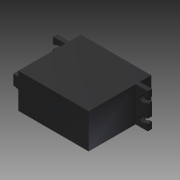
# Autodesk Inventor part: servo 4.8kg TGY-S4505B
Saved by Autodesk Inventor 2013 (Build 170138000, 138)
## iProperties
Created: 2013-03-06
Part Number: servo 4.8kg TGY-S4505B
Material: Generic
Document SubType Name: Modeling
Designer: Masta
Density: 1 g/cm^3
Author: Masta
Autodesk Inventor part; units mm, degrees
ref_plane "YZ Plane" through (0, 0, 0) normal (1, 0, 0) x (0, 1, 0)
ref_plane "XZ Plane" through (0, 0, 0) normal (0, 1, 0) x (-1, 0, 0)
ref_plane "XY Plane" through (0, 0, 0) normal (0, 0, 1) x (1, 0, 0)
sketch "Sketch1" plane through (0, 0, 0) normal (0, 1, 0) x (-1, 0, 0)
  line L0 (20.25, 10) -> (-20.25, 10)
  line L1 (-20.25, 10) -> (-20.25, -10)
  line L2 (-20.25, -10) -> (20.25, -10)
  line L3 (20.25, -10) -> (20.25, 10)
  line L4 (20.25, 10) -> (-20.25, -10) construction
  line L5 (-20.25, 10) -> (20.25, -10) construction
  line L6 (-27.25, 10) -> (-27.25, 6.25)
  line L7 (27.25, -10) -> (27.25, -6.25)
  line L8 (27.25, 10) -> (-27.25, -10) construction
  line L9 (-27.25, 10) -> (27.25, -10) construction
  line L10 (20.25, -10) -> (27.25, -10)
  line L11 (20.25, 10) -> (27.25, 10)
  line L12 (-20.25, 10) -> (-27.25, 10)
  line L13 (-20.25, -10) -> (-27.25, -10)
  line L14 (24.25, 5) -> (-24.25, 5) construction
  line L15 (-24.25, 5) -> (-24.25, -5) construction
  line L16 (-24.25, -5) -> (24.25, -5) construction
  line L17 (24.25, -5) -> (24.25, 5) construction
  line L18 (24.25, 5) -> (-24.25, -5) construction
  line L19 (-24.25, 5) -> (24.25, -5) construction
  circle A0 centre (-24.25, 5) radius 2
  line L20 (-27.25, 3.75) -> (-25.8112, 3.75)
  line L21 (-27.25, 6.25) -> (-25.8112, 6.25)
  line L22 (-20.25, 0) -> (20.25, 0) construction
  line L23 (0, 10) -> (0, -10) construction
  circle A1 centre (-24.25, -5) radius 2
  line L24 (-27.25, -3.75) -> (-25.8112, -3.75)
  line L25 (-27.25, -6.25) -> (-25.8112, -6.25)
  circle A2 centre (24.25, 5) radius 2
  line L26 (27.25, 3.75) -> (25.8112, 3.75)
  line L27 (27.25, 6.25) -> (25.8112, 6.25)
  line L28 (27.25, -6.25) -> (25.8112, -6.25)
  line L29 (27.25, -3.75) -> (25.8112, -3.75)
  circle A3 centre (24.25, -5) radius 2
  line L30 (-27.25, 3.75) -> (-27.25, -3.75)
  line L31 (-27.25, 6.25) -> (-27.25, 3.75)
  line L32 (-27.25, -6.25) -> (-27.25, -10)
  line L33 (-27.25, -3.75) -> (-27.25, -6.25)
  line L34 (27.25, -3.75) -> (27.25, 3.75)
  line L35 (27.25, -6.25) -> (27.25, -3.75)
  line L36 (27.25, 3.75) -> (27.25, 6.25)
  line L37 (27.25, 6.25) -> (27.25, 10)
  point P0 (0, 0)
  dimension "d0" = 40.5
  dimension "d1" = 20
  dimension "d2" = 54.5
  dimension "d3" = 48.5
  dimension "d4" = 10
  dimension "d12" = 2.5
  dimension "d13" = 4
  constraints: 76 end point, 32 parallel, 15 symmetric about line, 12 perpendicular, 10 midpoint, 8 point on circle, 4 centre point, 2 collinear, 2 horizontal, 1 coincident, 4 other
  measures "d0" distance of L2.end L1.end
  measures "d1" distance of L1.end L0.end
  measures "d2" distance of L7.start L8.end
  measures "d3" distance of L16.end L15.end
  measures "d4" distance of L15.end L14.end
  measures "d12" distance between parallel lines of L20 L21
  measures "d13" diameter of A0
extrude "Extrusion1" add sketch "Sketch1" along normal blind 9 and the other way blind 27 contours L3 L2 L1 L0
extrude "Extrusion2" add sketch "Sketch1" along normal blind 2.4 contours L11 L37 L27 A2 L26 L34 L29 A3 L28 L7 L10 L3 | L1 L13 L32 L25 A1 L24 L30 L20 A0 L21 L6 L12
sketch "Sketch2" plane through (0, 9, 0) normal (0, 1, 0) x (1, 0, 0)
  line L0 (-20.25, 10) -> (-20.25, -10) projected
  circle A0 centre (-10.25, 0) radius 7
  line L1 (-10.25, 0) -> (0, 0) construction
  dimension "d14" = 14
  dimension "d15" = 10
  constraints: 2 end point, 1 centre point, 1 perpendicular
  measures "d14" diameter of A0
  measures "d15" distance from line of L1.start L0
extrude "Extrusion3" add sketch "Sketch2" along normal blind 2
sketch "Sketch3" plane through (-10.25, 11, 0) normal (0, 1, 0) x (1, 0, 0)
  circle A0 centre (0, 0) radius 7 projected
  circle A1 centre (0, 0) radius 3
  point P0 (10.25, 0)
  dimension "d18" = 6
  constraints: 1 centre point, 1 coincident
  measures "d18" diameter of A1
extrude "Extrusion4" add sketch "Sketch3" along normal blind 4 contours A1
sketch "Sketch4" plane through (-20.25, -27, -10) normal (-1, 0, 0) x (0, 0, 1)
  line L0 (20, 27) -> (0, 27) projected
  line L1 (6.5, 3.5) -> (13.5, 3.5)
  line L2 (13.5, 3.5) -> (13.5, 8)
  line L3 (13.5, 8) -> (6.5, 8)
  line L4 (6.5, 8) -> (6.5, 3.5)
  line L5 (6.5, 3.5) -> (13.5, 8) construction
  line L6 (13.5, 3.5) -> (6.5, 8) construction
  line L7 (10, 27) -> (10, 5.75) construction
  dimension "d21" = 7
  dimension "d22" = 4.5
  dimension "d23" = 19
  constraints: 14 end point, 3 parallel, 2 midpoint, 1 horizontal, 1 perpendicular
  measures "d21" distance of L3.end L2.end
  measures "d22" distance of L2.end L1.end
  measures "d23" distance between parallel lines of L0 L3
extrude "Extrusion5" add sketch "Sketch4" along normal blind 7 draft -5
sketch "Sketch5" plane through (0, 0, 0) normal (0, 0, 1) x (1, 0, 0)
  line L0 (27.25, 2.4) -> (27.25, 0) projected
  line L1 (27.25, 0) -> (20.25, 0) projected
  line L2 (20.25, 0) -> (20.25, -27) projected
  line L3 (20.25, -27) -> (-20.25, -27) projected
  line L4 (-20.25, -23.5) -> (-27.25, -22.8876) projected
  line L5 (-27.25, -22.8876) -> (-27.25, -19.6124) projected
  line L6 (-27.25, -19.6124) -> (-20.25, -19) projected
  line L7 (-20.25, -19) -> (-20.25, 0) projected
  line L8 (-20.25, 0) -> (-27.25, 0) projected
  line L9 (-27.25, 0) -> (-27.25, 2.4) projected
  line L10 (-27.25, 2.4) -> (-20.25, 2.4) projected
  line L11 (-20.25, 2.4) -> (-20.25, 9) projected
  line L12 (-20.25, 9) -> (-17.25, 9) projected
  line L13 (-17.25, 9) -> (-17.25, 11) projected
  line L14 (-17.25, 11) -> (-13.25, 11) projected
  line L15 (-13.25, 11) -> (-13.25, 15) projected
  line L16 (-13.25, 15) -> (-7.25, 15) projected
  line L17 (-7.25, 15) -> (-7.25, 11) projected
  line L18 (-7.25, 11) -> (-3.25, 11) projected
  line L19 (-3.25, 11) -> (-3.25, 9) projected
  line L20 (-3.25, 9) -> (20.25, 9) projected
  line L21 (20.25, 9) -> (20.25, 2.4) projected
  line L22 (20.25, 2.4) -> (27.25, 2.4) projected
  line L23 (-27.25, 2.4) -> (-20.25, 3.5)
  line L24 (20.25, 3.5) -> (27.25, 2.4)
  line L25 (-20.25, -27) -> (-20.25, -23.5) projected
  point P0 (0, 0)
  dimension "d26" = 1.1
  constraints: 4 end point, 2 point on line, 1 equal length
  measures "d26" distance of L23.end L10.end
extrude "Extrusion6" add sketch "Sketch5" along normal mid plane 1.3 contours L22 L21 L24 | L23 L11 L10
sketch "Sketch6" plane through (0, 9, 0) normal (0, 1, 0) x (1, 0, 0)
  line L0 (12.3297, -9.4801) -> (12.3297, 4.6475) construction
  line L1 (12.3297, 4.6475) -> (15.9034, 4.6475) construction
  line L2 (15.9034, 4.6475) -> (15.9034, -9.4801) construction
  line L3 (15.9034, -9.4801) -> (12.3297, -9.4801) construction
  line L4 (14.8526, -8.6525) -> (12.6724, -8.6525)
  line L5 (12.6724, -8.6525) -> (12.6724, -9.4821)
  line L6 (12.6724, -9.4821) -> (12.3798, -9.4821)
  line L7 (12.3798, -9.4821) -> (12.3798, -7.4942)
  line L8 (12.3798, -7.4942) -> (12.6724, -7.4942)
  line L9 (12.6724, -7.4942) -> (12.6724, -8.3238)
  line L10 (12.6724, -8.3238) -> (14.8526, -8.3238)
  line L11 (14.8526, -8.3238) -> (14.8526, -8.6525)
  spline S0 degree 2 poles (14.9007, -6.2077) (14.9007, -6.4702) (14.7404, -6.9051) (14.5781, -7.0614) knots 0 0 0 1 2 2 2
  spline S1 degree 2 poles (14.5781, -7.0614) (14.4137, -7.2177) (13.9288, -7.384) (13.6142, -7.384) knots 0 0 0 1 2 2 2
  spline S2 degree 2 poles (13.6142, -7.384) (13.3156, -7.384) (12.8427, -7.2157) (12.6744, -7.0594) knots 0 0 0 1 2 2 2
  spline S3 degree 2 poles (12.6744, -7.0594) (12.512, -6.9091) (12.3357, -6.4682) (12.3357, -6.2057) knots 0 0 0 1 2 2 2
  spline S4 degree 2 poles (12.3357, -6.2057) (12.3357, -6.0795) (12.3718, -5.851) (12.4038, -5.7468) knots 0 0 0 1 2 2 2
  spline S5 degree 2 poles (12.4038, -5.7468) (12.4279, -5.6627) (12.516, -5.4583) (12.5481, -5.3961) knots 0 0 0 1 2 2 2
  line L12 (12.5481, -5.3961) -> (12.9449, -5.3961)
  line L13 (12.9449, -5.3961) -> (12.9449, -5.4242)
  spline S6 degree 2 poles (12.9449, -5.4242) (12.8908, -5.4863) (12.7926, -5.6166) (12.7365, -5.7368) knots 0 0 0 1 2 2 2
  spline S7 degree 2 poles (12.7365, -5.7368) (12.6864, -5.837) (12.6202, -6.0955) (12.6202, -6.2438) knots 0 0 0 1 2 2 2
  spline S8 degree 2 poles (12.6202, -6.2438) (12.6202, -6.6005) (13.1573, -7.0413) (13.6042, -7.0413) knots 0 0 0 1 2 2 2
  spline S9 degree 2 poles (13.6042, -7.0413) (13.8527, -7.0413) (14.2254, -6.9251) (14.3536, -6.8149) knots 0 0 0 1 2 2 2
  spline S10 degree 2 poles (14.3536, -6.8149) (14.4819, -6.7087) (14.6161, -6.4081) (14.6161, -6.2197) knots 0 0 0 1 2 2 2
  spline S11 degree 2 poles (14.6161, -6.2197) (14.6161, -6.0815) (14.5761, -5.8049) (14.536, -5.7107) knots 0 0 0 1 2 2 2
  line L14 (14.536, -5.7107) -> (13.8967, -5.7107)
  line L15 (13.8967, -5.7107) -> (13.8967, -6.2839)
  line L16 (13.8967, -6.2839) -> (13.6082, -6.2839)
  line L17 (13.6082, -6.2839) -> (13.6082, -5.3861)
  line L18 (13.6082, -5.3861) -> (14.6883, -5.3861)
  spline S12 degree 2 poles (14.6883, -5.3861) (14.7163, -5.4482) (14.8025, -5.6607) (14.8286, -5.7508) knots 0 0 0 1 2 2 2
  spline S13 degree 2 poles (14.8286, -5.7508) (14.8646, -5.8731) (14.9007, -6.0694) (14.9007, -6.2077) knots 0 0 0 1 2 2 2
  line L19 (12.3798, -3.2419) -> (13.7585, -4.0776)
  line L20 (13.7585, -4.0776) -> (14.8526, -4.0776)
  line L21 (14.8526, -4.0776) -> (14.8526, -4.4062)
  line L22 (14.8526, -4.4062) -> (13.7925, -4.4062)
  line L23 (13.7925, -4.4062) -> (12.3798, -5.2418)
  line L24 (12.3798, -5.2418) -> (12.3798, -4.8771)
  line L25 (12.3798, -4.8771) -> (13.4679, -4.2399)
  line L26 (13.4679, -4.2399) -> (12.3798, -3.5906)
  line L27 (12.3798, -3.5906) -> (12.3798, -3.2419)
  line L28 (13.9208, -2.1779) -> (13.9208, -3.1137)
  line L29 (13.9208, -3.1137) -> (13.6202, -3.1137)
  line L30 (13.6202, -3.1137) -> (13.6202, -2.1779)
  line L31 (13.6202, -2.1779) -> (13.9208, -2.1779)
  spline S14 degree 2 poles (14.8967, -1.0897) (14.8967, -1.3583) (14.7845, -1.735) (14.7043, -1.9013) knots 0 0 0 1 2 2 2
  line L32 (14.7043, -1.9013) -> (14.2915, -1.9013)
  line L33 (14.2915, -1.9013) -> (14.2915, -1.8773)
  spline S15 degree 2 poles (14.2915, -1.8773) (14.4438, -1.715) (14.6121, -1.3041) (14.6121, -1.1138) knots 0 0 0 1 2 2 2
  spline S16 degree 2 poles (14.6121, -1.1138) (14.6121, -0.8412) (14.3857, -0.5627) (14.1993, -0.5627) knots 0 0 0 1 2 2 2
  spline S17 degree 2 poles (14.1993, -0.5627) (14.051, -0.5627) (13.8667, -0.709) (13.8206, -0.8673) knots 0 0 0 1 2 2 2
  spline S18 degree 2 poles (13.8206, -0.8673) (13.7885, -0.9815) (13.7444, -1.1719) (13.7084, -1.3142) knots 0 0 0 1 2 2 2
  spline S19 degree 2 poles (13.7084, -1.3142) (13.6743, -1.4424) (13.5721, -1.6448) (13.4899, -1.723) knots 0 0 0 1 2 2 2
  spline S20 degree 2 poles (13.4899, -1.723) (13.4078, -1.7991) (13.1874, -1.8833) (13.0431, -1.8833) knots 0 0 0 1 2 2 2
  spline S21 degree 2 poles (13.0431, -1.8833) (12.7425, -1.8833) (12.3357, -1.4144) (12.3357, -1.0517) knots 0 0 0 1 2 2 2
  spline S22 degree 2 poles (12.3357, -1.0517) (12.3357, -0.8433) (12.4179, -0.4745) (12.496, -0.3162) knots 0 0 0 1 2 2 2
  line L34 (12.496, -0.3162) -> (12.8888, -0.3162)
  line L35 (12.8888, -0.3162) -> (12.8888, -0.3403)
  spline S23 degree 2 poles (12.8888, -0.3403) (12.7806, -0.4585) (12.6202, -0.8272) (12.6202, -1.0296) knots 0 0 0 1 2 2 2
  spline S24 degree 2 poles (12.6202, -1.0296) (12.6202, -1.2581) (12.8347, -1.5406) (13.009, -1.5406) knots 0 0 0 1 2 2 2
  spline S25 degree 2 poles (13.009, -1.5406) (13.1653, -1.5406) (13.3517, -1.3743) (13.3938, -1.218) knots 0 0 0 1 2 2 2
  spline S26 degree 2 poles (13.3938, -1.218) (13.4218, -1.1138) (13.494, -0.8112) (13.524, -0.711) knots 0 0 0 1 2 2 2
  spline S27 degree 2 poles (13.524, -0.711) (13.6022, -0.4565) (13.9168, -0.22) (14.1472, -0.22) knots 0 0 0 1 2 2 2
  spline S28 degree 2 poles (14.1472, -0.22) (14.2935, -0.22) (14.5741, -0.3383) (14.6723, -0.4445) knots 0 0 0 1 2 2 2
  spline S29 degree 2 poles (14.6723, -0.4445) (14.7805, -0.5627) (14.8967, -0.8633) (14.8967, -1.0897) knots 0 0 0 1 2 2 2
  line L36 (14.0029, 1.6356) -> (14.0029, 1.341)
  line L37 (14.0029, 1.341) -> (14.8526, 1.341)
  line L38 (14.8526, 1.341) -> (14.8526, 1.0224)
  line L39 (14.8526, 1.0224) -> (14.0029, 1.0224)
  line L40 (14.0029, 1.0224) -> (14.0029, -0.0697)
  line L41 (14.0029, -0.0697) -> (13.6543, -0.0697)
  line L42 (13.6543, -0.0697) -> (12.3798, 1.0364)
  line L43 (12.3798, 1.0364) -> (12.3798, 1.341)
  line L44 (12.3798, 1.341) -> (13.7364, 1.341)
  line L45 (13.7364, 1.341) -> (13.7364, 1.6356)
  line L46 (13.7364, 1.6356) -> (14.0029, 1.6356)
  line L47 (13.7364, 1.0224) -> (12.7705, 1.0224)
  line L48 (12.7705, 1.0224) -> (13.7364, 0.1908)
  line L49 (13.7364, 0.1908) -> (13.7364, 1.0224)
  spline S30 degree 2 poles (14.0671, 3.399) (14.2454, 3.399) (14.55, 3.2848) (14.6622, 3.1806) knots 0 0 0 1 2 2 2
  spline S31 degree 2 poles (14.6622, 3.1806) (14.7745, 3.0764) (14.9047, 2.7658) (14.9047, 2.5734) knots 0 0 0 1 2 2 2
  spline S32 degree 2 poles (14.9047, 2.5734) (14.9047, 2.3971) (14.8266, 2.0524) (14.7644, 1.9262) knots 0 0 0 1 2 2 2
  line L50 (14.7644, 1.9262) -> (14.4137, 1.9262)
  line L51 (14.4137, 1.9262) -> (14.4137, 1.9502)
  spline S33 degree 2 poles (14.4137, 1.9502) (14.4418, 1.9883) (14.5139, 2.1306) (14.546, 2.2167) knots 0 0 0 1 2 2 2
  spline S34 degree 2 poles (14.546, 2.2167) (14.5801, 2.3149) (14.6181, 2.4772) (14.6181, 2.5794) knots 0 0 0 1 2 2 2
  spline S35 degree 2 poles (14.6181, 2.5794) (14.6181, 2.6796) (14.546, 2.868) (14.4679, 2.9361) knots 0 0 0 1 2 2 2
  spline S36 degree 2 poles (14.4679, 2.9361) (14.3937, 2.9982) (14.1973, 3.0624) (14.0651, 3.0624) knots 0 0 0 1 2 2 2
  spline S37 degree 2 poles (14.0651, 3.0624) (13.9328, 3.0624) (13.7645, 2.9902) (13.7084, 2.9221) knots 0 0 0 1 2 2 2
  spline S38 degree 2 poles (13.7084, 2.9221) (13.6463, 2.852) (13.5942, 2.6436) (13.5942, 2.5173) knots 0 0 0 1 2 2 2
  spline S39 degree 2 poles (13.5942, 2.5173) (13.5942, 2.381) (13.6362, 2.1105) (13.6543, 2.0284) knots 0 0 0 1 2 2 2
  line L52 (13.6543, 2.0284) -> (12.3798, 2.0284)
  line L53 (12.3798, 2.0284) -> (12.3798, 3.385)
  line L54 (12.3798, 3.385) -> (12.6703, 3.385)
  line L55 (12.6703, 3.385) -> (12.6703, 2.347)
  line L56 (12.6703, 2.347) -> (13.3296, 2.347)
  spline S40 degree 2 poles (13.3296, 2.347) (13.3216, 2.4071) (13.3156, 2.5233) (13.3156, 2.5714) knots 0 0 0 1 2 2 2
  spline S41 degree 2 poles (13.3156, 2.5714) (13.3156, 2.7618) (13.3777, 3.0243) (13.4699, 3.1445) knots 0 0 0 1 2 2 2
  spline S42 degree 2 poles (13.4699, 3.1445) (13.5621, 3.2668) (13.8426, 3.399) (14.0671, 3.399) knots 0 0 0 1 2 2 2
  spline S43 degree 2 poles (13.6162, 5.2947) (14.2815, 5.2947) (14.9047, 4.908) (14.9047, 4.5052) knots 0 0 0 1 2 2 2
  spline S44 degree 2 poles (14.9047, 4.5052) (14.9047, 4.0964) (14.2695, 3.7136) (13.6182, 3.7136) knots 0 0 0 1 2 2 2
  spline S45 degree 2 poles (13.6182, 3.7136) (12.9489, 3.7136) (12.3297, 4.1004) (12.3297, 4.5052) knots 0 0 0 1 2 2 2
  spline S46 degree 2 poles (12.3297, 4.5052) (12.3297, 4.912) (12.9709, 5.2947) (13.6162, 5.2947) knots 0 0 0 1 2 2 2
  spline S47 degree 2 poles (14.3697, 4.8699) (14.2474, 4.918) (13.8707, 4.9581) (13.6162, 4.9581) knots 0 0 0 1 2 2 2
  spline S48 degree 2 poles (13.6162, 4.9581) (13.3617, 4.9581) (12.987, 4.918) (12.8607, 4.8679) knots 0 0 0 1 2 2 2
  spline S49 degree 2 poles (12.8607, 4.8679) (12.7345, 4.8178) (12.6042, 4.6435) (12.6042, 4.5052) knots 0 0 0 1 2 2 2
  spline S50 degree 2 poles (12.6042, 4.5052) (12.6042, 4.3669) (12.7345, 4.1886) (12.8647, 4.1365) knots 0 0 0 1 2 2 2
  spline S51 degree 2 poles (12.8647, 4.1365) (12.991, 4.0864) (13.3757, 4.0503) (13.6182, 4.0503) knots 0 0 0 1 2 2 2
  spline S52 degree 2 poles (13.6182, 4.0503) (13.8787, 4.0503) (14.2274, 4.0824) (14.3637, 4.1345) knots 0 0 0 1 2 2 2
  spline S53 degree 2 poles (14.3637, 4.1345) (14.4919, 4.1826) (14.6302, 4.3609) (14.6302, 4.5052) knots 0 0 0 1 2 2 2
  spline S54 degree 2 poles (14.6302, 4.5052) (14.6302, 4.6415) (14.4999, 4.8198) (14.3697, 4.8699) knots 0 0 0 1 2 2 2
  spline S55 degree 2 poles (14.0671, 7.1103) (14.2454, 7.1103) (14.55, 6.996) (14.6622, 6.8918) knots 0 0 0 1 2 2 2
  spline S56 degree 2 poles (14.6622, 6.8918) (14.7745, 6.7876) (14.9047, 6.477) (14.9047, 6.2847) knots 0 0 0 1 2 2 2
  spline S57 degree 2 poles (14.9047, 6.2847) (14.9047, 6.1083) (14.8266, 5.7636) (14.7644, 5.6374) knots 0 0 0 1 2 2 2
  line L57 (14.7644, 5.6374) -> (14.4137, 5.6374)
  line L58 (14.4137, 5.6374) -> (14.4137, 5.6614)
  spline S58 degree 2 poles (14.4137, 5.6614) (14.4418, 5.6995) (14.5139, 5.8418) (14.546, 5.928) knots 0 0 0 1 2 2 2
  spline S59 degree 2 poles (14.546, 5.928) (14.5801, 6.0262) (14.6181, 6.1885) (14.6181, 6.2907) knots 0 0 0 1 2 2 2
  spline S60 degree 2 poles (14.6181, 6.2907) (14.6181, 6.3909) (14.546, 6.5792) (14.4679, 6.6474) knots 0 0 0 1 2 2 2
  spline S61 degree 2 poles (14.4679, 6.6474) (14.3937, 6.7095) (14.1973, 6.7736) (14.0651, 6.7736) knots 0 0 0 1 2 2 2
  spline S62 degree 2 poles (14.0651, 6.7736) (13.9328, 6.7736) (13.7645, 6.7015) (13.7084, 6.6333) knots 0 0 0 1 2 2 2
  spline S63 degree 2 poles (13.7084, 6.6333) (13.6463, 6.5632) (13.5942, 6.3548) (13.5942, 6.2286) knots 0 0 0 1 2 2 2
  spline S64 degree 2 poles (13.5942, 6.2286) (13.5942, 6.0923) (13.6362, 5.8218) (13.6543, 5.7396) knots 0 0 0 1 2 2 2
  line L59 (13.6543, 5.7396) -> (12.3798, 5.7396)
  line L60 (12.3798, 5.7396) -> (12.3798, 7.0962)
  line L61 (12.3798, 7.0962) -> (12.6703, 7.0962)
  line L62 (12.6703, 7.0962) -> (12.6703, 6.0582)
  line L63 (12.6703, 6.0582) -> (13.3296, 6.0582)
  spline S65 degree 2 poles (13.3296, 6.0582) (13.3216, 6.1183) (13.3156, 6.2346) (13.3156, 6.2827) knots 0 0 0 1 2 2 2
  spline S66 degree 2 poles (13.3156, 6.2827) (13.3156, 6.473) (13.3777, 6.7355) (13.4699, 6.8558) knots 0 0 0 1 2 2 2
  spline S67 degree 2 poles (13.4699, 6.8558) (13.5621, 6.978) (13.8426, 7.1103) (14.0671, 7.1103) knots 0 0 0 1 2 2 2
  spline S68 degree 2 poles (14.0931, 9.2144) (14.2775, 9.2144) (14.56, 9.0741) (14.6522, 8.9579) knots 0 0 0 1 2 2 2
  spline S69 degree 2 poles (14.6522, 8.9579) (14.7604, 8.8176) (14.8526, 8.499) (14.8526, 8.2465) knots 0 0 0 1 2 2 2
  line L64 (14.8526, 8.2465) -> (14.8526, 7.5371)
  line L65 (14.8526, 7.5371) -> (12.3798, 7.5371)
  line L66 (12.3798, 7.5371) -> (12.3798, 8.1924)
  spline S70 degree 2 poles (12.3798, 8.1924) (12.3798, 8.4569) (12.4138, 8.7214) (12.48, 8.8417) knots 0 0 0 1 2 2 2
  spline S71 degree 2 poles (12.48, 8.8417) (12.5501, 8.9759) (12.7806, 9.0982) (12.9369, 9.0982) knots 0 0 0 1 2 2 2
  spline S72 degree 2 poles (12.9369, 9.0982) (13.1112, 9.0982) (13.3877, 8.9138) (13.4659, 8.7515) knots 0 0 0 1 2 2 2
  line L67 (13.4659, 8.7515) -> (13.4779, 8.7515)
  spline S73 degree 2 poles (13.4779, 8.7515) (13.538, 8.9719) (13.8567, 9.2144) (14.0931, 9.2144) knots 0 0 0 1 2 2 2
  spline S74 degree 2 poles (14.1072, 8.8717) (13.9669, 8.8717) (13.7865, 8.7916) (13.7224, 8.6713) knots 0 0 0 1 2 2 2
  spline S75 degree 2 poles (13.7224, 8.6713) (13.6823, 8.5932) (13.6583, 8.4088) (13.6583, 8.2385) knots 0 0 0 1 2 2 2
  line L68 (13.6583, 8.2385) -> (13.6583, 7.8657)
  line L69 (13.6583, 7.8657) -> (14.5721, 7.8657)
  line L70 (14.5721, 7.8657) -> (14.5721, 8.1323)
  spline S76 degree 2 poles (14.5721, 8.1323) (14.5721, 8.3487) (14.532, 8.5972) (14.4679, 8.6934) knots 0 0 0 1 2 2 2
  spline S77 degree 2 poles (14.4679, 8.6934) (14.4017, 8.7855) (14.2374, 8.8717) (14.1072, 8.8717) knots 0 0 0 1 2 2 2
  spline S78 degree 2 poles (12.983, 8.7555) (12.8948, 8.7555) (12.7625, 8.6954) (12.7245, 8.6292) knots 0 0 0 1 2 2 2
  spline S79 degree 2 poles (12.7245, 8.6292) (12.6804, 8.5491) (12.6603, 8.3547) (12.6603, 8.1804) knots 0 0 0 1 2 2 2
  line L71 (12.6603, 8.1804) -> (12.6603, 7.8657)
  line L72 (12.6603, 7.8657) -> (13.3837, 7.8657)
  line L73 (13.3837, 7.8657) -> (13.3837, 8.2385)
  spline S80 degree 2 poles (13.3837, 8.2385) (13.3837, 8.3928) (13.3517, 8.5391) (13.3016, 8.6172) knots 0 0 0 1 2 2 2
  spline S81 degree 2 poles (13.3016, 8.6172) (13.2535, 8.6934) (13.0992, 8.7555) (12.983, 8.7555) knots 0 0 0 1 2 2 2
  point P0 (0, 0)
  constraints: 2 other
emboss "Emboss1" sketch "Sketch6" operation cut depth 0.1 direction (0, -1, 0)
hole "Hole1" at (-10.25, 15, 0) direction (0, -1, 0) diameter 2.459 depth 8 tip angle 118 thread size "M3x0.5" class "6H" standard "ISO Metric profile"
body "Solid1"
